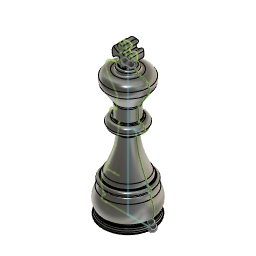
King v1 (Autodesk Fusion 360 design; units mm, degrees)
Autodesk Fusion 360 part; units mm, degrees
sketch "Sketch1" plane through (0, 0, 0) normal (0, 1, 0) x (1, 0, 0)
  spline S0 degree 3 poles (-2.3239, -43.7499) (-1.9635, -43.3416) (-1.5711, -43.0534) (-1.0977, -42.8653) knots 0 0 0 0 1 1 1 1
  spline S1 degree 3 poles (-1.0977, -42.8653) (-0.9162, -42.7932) (-0.7519, -42.7656) (-0.5988, -42.8557) knots 0 0 0 0 1 1 1 1
  spline S2 degree 3 poles (-0.5988, -42.8557) (-0.387, -42.9817) (-0.4437, -43.2144) (-0.4862, -43.3933) knots 0 0 0 0 1 1 1 1
  spline S3 degree 3 poles (-0.4862, -43.3933) (-0.5788, -43.7825) (-0.7682, -44.124) (-1.0818, -44.3926) knots 0 0 0 0 1 1 1 1
  spline S4 degree 3 poles (-1.0818, -44.3926) (-1.35, -44.6225) (-1.2716, -44.7951) (-0.9684, -44.9232) knots 0 0 0 0 1 1 1 1
  spline S5 degree 3 poles (-0.9684, -44.9232) (-0.5113, -45.1159) (-0.0212, -45.1676) (0.4476, -45.1021) knots 0 0 0 0 1 1 1 1
  spline S6 degree 3 poles (0.4476, -45.1021) (1.3114, -44.9807) (1.3468, -44.8256) (0.848, -44.1249) knots 0 0 0 0 1 1 1 1
  spline S7 degree 3 poles (0.848, -44.1249) (0.6019, -43.7791) (0.1882, -43.357) (0.5857, -42.9642) knots 0 0 0 0 1 1 1 1
  spline S8 degree 3 poles (0.5857, -42.9642) (1.0165, -42.5379) (1.4507, -42.9996) (1.7956, -43.2557) knots 0 0 0 0 1 1 1 1
  spline S9 degree 3 poles (1.7956, -43.2557) (2.3849, -43.6932) (2.5622, -43.6807) (2.6819, -42.9725) knots 0 0 0 0 1 1 1 1
  spline S10 degree 3 poles (2.6819, -42.9725) (2.7753, -42.4182) (2.8325, -41.8455) (2.5668, -41.2929) knots 0 0 0 0 1 1 1 1
  spline S11 degree 3 poles (2.5668, -41.2929) (2.4133, -40.9738) (2.3132, -40.8383) (2.0379, -41.1878) knots 0 0 0 0 1 1 1 1
  spline S12 degree 3 poles (2.0379, -41.1878) (1.7877, -41.5044) (1.4382, -41.7092) (1.0528, -41.8168) knots 0 0 0 0 1 1 1 1
  spline S13 degree 3 poles (1.0528, -41.8168) (0.5973, -41.9436) (0.3763, -41.7179) (0.4718, -41.257) knots 0 0 0 0 1 1 1 1
  spline S14 degree 3 poles (0.4718, -41.257) (0.5652, -40.807) (0.8701, -40.4804) (1.1433, -40.1389) knots 0 0 0 0 1 1 1 1
  spline S15 degree 3 poles (1.1433, -40.1389) (1.3568, -39.8719) (1.331, -39.7493) (0.9702, -39.6563) knots 0 0 0 0 1 1 1 1
  spline S16 degree 3 poles (-0.842, -39.6271) (-1.2416, -39.7656) (-1.4835, -39.9145) (-1.0451, -40.3378) knots 0 0 0 0 1 1 1 1
  spline S17 degree 3 poles (-1.0451, -40.3378) (-0.8024, -40.5722) (-0.6643, -40.9205) (-0.5012, -41.2291) knots 0 0 0 0 1 1 1 1
  spline S18 degree 3 poles (-0.5012, -41.2291) (-0.4137, -41.3951) (-0.4491, -41.5836) (-0.5747, -41.7225) knots 0 0 0 0 1 1 1 1
  spline S19 degree 3 poles (-0.5747, -41.7225) (-0.7056, -41.8677) (-0.8674, -41.8681) (-1.0539, -41.7888) knots 0 0 0 0 1 1 1 1
  spline S20 degree 3 poles (-1.0539, -41.7888) (-1.4343, -41.627) (-1.8321, -41.5044) (-2.1103, -41.1678) knots 0 0 0 0 1 1 1 1
  spline S21 degree 3 poles (-2.1103, -41.1678) (-2.3314, -40.9004) (-2.474, -41.0022) (-2.562, -41.2804) knots 0 0 0 0 1 1 1 1
  spline S22 degree 3 poles (-2.562, -41.2804) (-2.8227, -42.1058) (-2.8648, -42.9133) (-2.3239, -43.7499) knots 0 0 0 0 1 1 1 1
  spline S23 degree 3 poles (5.7912, -10.8328) (5.8309, -11.2607) (5.5652, -11.6023) (5.3888, -11.9368) knots 0 0 0 0 1 1 1 1
  spline S24 degree 3 poles (5.3888, -11.9368) (3.7392, -15.0636) (2.7616, -18.3765) (2.5151, -21.9046) knots 0 0 0 0 1 1 1 1
  spline S25 degree 3 poles (2.5151, -21.9046) (2.4513, -22.82) (2.4329, -22.9965) (1.829, -23.074) knots 0 0 0 0 1 1 1 1
  spline S26 degree 3 poles (-2.4465, -23.074) (-2.5929, -23.0336) (-2.7093, -22.9377) (-2.7105, -22.7053) knots 0 0 0 0 1 1 1 1
  spline S27 degree 3 poles (-2.7105, -22.7053) (-2.7118, -22.3537) (-2.8273, -22.0076) (-2.834, -21.6718) knots 0 0 0 0 1 1 1 1
  spline S28 degree 3 poles (-2.834, -21.6718) (-2.8707, -19.8429) (-3.2556, -18.0758) (-3.6952, -16.3157) knots 0 0 0 0 1 1 1 1
  spline S29 degree 3 poles (-3.6952, -16.3157) (-4.1136, -14.6415) (-4.9444, -13.1288) (-5.5825, -11.541) knots 0 0 0 0 1 1 1 1
  spline S30 degree 3 poles (-5.5825, -11.541) (-5.6889, -11.2765) (-5.8736, -11.01) (-5.6901, -10.8328) knots 0 0 0 0 1 1 1 1
  spline S31 degree 3 poles (6.366, -9.2437) (6.6016, -9.3409) (6.7555, -9.5569) (6.8002, -9.828) knots 0 0 0 0 1 1 1 1
  spline S32 degree 3 poles (6.8002, -9.828) (6.8594, -10.1917) (6.5028, -10.4661) (6.102, -10.5763) knots 0 0 0 0 1 1 1 1
  spline S33 degree 3 poles (6.102, -10.5763) (6.0519, -10.5904) (5.9789, -10.5842) (5.9155, -10.5959) knots 0 0 0 0 1 1 1 1
  spline S34 degree 3 poles (-5.9775, -10.5959) (-5.9883, -10.5946) (-5.9996, -10.5942) (-6.0109, -10.5934) knots 0 0 0 0 1 1 1 1
  spline S35 degree 3 poles (-6.0109, -10.5934) (-6.4855, -10.5642) (-6.7612, -10.2876) (-6.7478, -9.8372) knots 0 0 0 0 1 1 1 1
  spline S36 degree 3 poles (-6.7478, -9.8372) (-6.737, -9.4914) (-6.5443, -9.3062) (-6.2461, -9.2437) knots 0 0 0 0 1 1 1 1
  spline S37 degree 3 poles (6.5778, -2.1049) (6.8669, -2.1729) (7.0758, -2.3423) (7.2439, -2.6838) knots 0 0 0 0 1 1 1 1
  spline S38 degree 3 poles (7.2439, -2.6838) (8.1119, -4.4448) (7.8479, -6.1373) (6.9599, -7.7785) knots 0 0 0 0 1 1 1 1
  spline S39 degree 3 poles (6.9599, -7.7785) (6.7297, -8.2039) (6.6129, -8.7857) (6.1437, -9.0068) knots 0 0 0 0 1 1 1 1
  spline S40 degree 3 poles (-2.7568, -9.0068) (-3.2202, -8.9926) (-3.6831, -8.9843) (-4.1428, -9.0068) knots 0 0 0 0 1 1 1 1
  line L0 (-4.1428, -9.0068) -> (-5.7452, -9.0068)
  spline S41 degree 3 poles (-5.7452, -9.0068) (-6.4004, -8.847) (-6.8692, -8.4024) (-7.2763, -7.6358) knots 0 0 0 0 1 1 1 1
  spline S42 degree 3 poles (-7.2763, -7.6358) (-8.1884, -5.9179) (-8.2602, -4.275) (-7.4014, -2.5525) knots 0 0 0 0 1 1 1 1
  spline S43 degree 3 poles (-7.4014, -2.5525) (-7.2792, -2.306) (-7.1278, -2.1675) (-6.9247, -2.1049) knots 0 0 0 0 1 1 1 1
  spline S44 degree 3 poles (-6.9426, -1.8693) (-7.5245, -1.7588) (-7.914, -1.2391) (-7.8143, -0.5701) knots 0 0 0 0 1 1 1 1
  spline S45 degree 3 poles (-7.8143, -0.5701) (-7.7167, 0.0906) (-7.1353, -0.3253) (-6.7766, -0.2389) knots 0 0 0 0 1 1 1 1
  spline S46 degree 3 poles (-6.7766, -0.2389) (-6.6736, -0.2131) (-6.5589, -0.2335) (-6.4492, -0.2335) knots 0 0 0 0 1 1 1 1
  spline S47 degree 3 poles (-6.4492, -0.2335) (-2.0686, -0.2322) (2.3128, -0.2264) (6.6938, -0.2464) knots 0 0 0 0 1 1 1 1
  spline S48 degree 3 poles (6.6938, -0.2464) (6.9666, -0.2477) (7.3691, -0.0512) (7.528, -0.4012) knots 0 0 0 0 1 1 1 1
  spline S49 degree 3 poles (7.528, -0.4012) (7.6906, -0.7586) (7.4992, -1.1227) (7.3102, -1.4572) knots 0 0 0 0 1 1 1 1
  spline S50 degree 3 poles (7.3102, -1.4572) (7.1684, -1.7079) (6.9774, -1.8205) (6.7543, -1.8693) knots 0 0 0 0 1 1 1 1
  spline S51 degree 3 poles (6.0999, -34.4728) (6.4285, -35.0642) (6.4552, -35.692) (6.2659, -36.3197) knots 0 0 0 0 1 1 1 1
  spline S52 degree 3 poles (6.2659, -36.3197) (5.9318, -37.4258) (5.0426, -37.988) (3.7179, -37.9513) knots 0 0 0 0 1 1 1 1
  spline S53 degree 3 poles (3.7179, -37.9513) (3.1649, -37.9354) (2.679, -37.9717) (2.7165, -38.7141) knots 0 0 0 0 1 1 1 1
  spline S54 degree 3 poles (2.7165, -38.7141) (2.7353, -39.0887) (2.4713, -39.2292) (2.1835, -39.23) knots 0 0 0 0 1 1 1 1
  spline S55 degree 3 poles (2.1835, -39.23) (0.7237, -39.235) (-0.7361, -39.2063) (-2.1963, -39.1975) knots 0 0 0 0 1 1 1 1
  spline S56 degree 3 poles (-2.1963, -39.1975) (-2.5629, -39.195) (-2.9366, -39.087) (-2.9495, -38.7137) knots 0 0 0 0 1 1 1 1
  spline S57 degree 3 poles (-2.9495, -38.7137) (-2.9716, -38.0731) (-3.2319, -37.8887) (-3.825, -37.9972) knots 0 0 0 0 1 1 1 1
  spline S58 degree 3 poles (-3.825, -37.9972) (-4.0114, -38.0318) (-4.2162, -37.9746) (-4.411, -37.9542) knots 0 0 0 0 1 1 1 1
  spline S59 degree 3 poles (-4.411, -37.9542) (-6.5343, -37.7336) (-7.162, -35.752) (-6.1794, -34.102) knots 0 0 0 0 1 1 1 1
  spline S60 degree 3 poles (-6.1794, -34.102) (-5.3281, -32.6731) (-4.3413, -31.3251) (-3.4129, -29.9421) knots 0 0 0 0 1 1 1 1
  spline S61 degree 3 poles (-3.4129, -29.9421) (-3.2715, -29.7315) (-3.231, -29.5079) (-3.2473, -29.2543) knots 0 0 0 0 1 1 1 1
  spline S62 degree 3 poles (-3.2473, -29.2543) (-3.3132, -28.2487) (-3.3741, -27.2436) (-3.4133, -26.2372) knots 0 0 0 0 1 1 1 1
  spline S63 degree 3 poles (-3.4133, -26.2372) (-3.4204, -26.0591) (-3.4437, -25.9227) (-3.5092, -25.8251) knots 0 0 0 0 1 1 1 1
  line L1 (-3.5092, -25.8251) -> (-4.0781, -25.8251)
  spline S64 degree 3 poles (-4.0781, -25.8251) (-4.7726, -25.8251) (-5.3356, -25.2625) (-5.3356, -24.5684) knots 0 0 0 0 1 1 1 1
  spline S65 degree 3 poles (-5.3356, -24.5684) (-5.3356, -23.9378) (-4.8714, -23.4177) (-4.2666, -23.3268) knots 0 0 0 0 1 1 1 1
  spline S66 degree 3 poles (-4.2666, -23.3268) (-4.2479, -23.3222) (-4.2308, -23.3155) (-4.212, -23.3114) knots 0 0 0 0 1 1 1 1
  line L2 (-4.212, -23.3114) -> (-4.0781, -23.3114)
  line L3 (3.7338, -23.3114) -> (3.9056, -23.3114)
  spline S67 degree 3 poles (3.9056, -23.3114) (4.1555, -23.3593) (4.3632, -23.4552) (4.5237, -23.5912) knots 0 0 0 0 1 1 1 1
  spline S68 degree 3 poles (4.5237, -23.5912) (4.5287, -23.5946) (4.5333, -23.5987) (4.5383, -23.6025) knots 0 0 0 0 1 1 1 1
  spline S69 degree 3 poles (4.5383, -23.6025) (4.555, -23.6175) (4.5721, -23.6317) (4.5875, -23.6475) knots 0 0 0 0 1 1 1 1
  spline S70 degree 3 poles (4.5875, -23.6475) (4.8353, -23.8769) (4.9909, -24.2039) (4.9909, -24.5684) knots 0 0 0 0 1 1 1 1
  spline S71 degree 3 poles (4.9909, -24.5684) (4.9909, -25.2625) (4.4278, -25.8251) (3.7338, -25.8251) knots 0 0 0 0 1 1 1 1
  line L4 (3.7338, -25.8251) -> (3.275, -25.8251)
  spline S72 degree 3 poles (3.275, -25.8251) (3.2262, -25.8872) (3.1995, -25.9727) (3.1949, -26.0924) knots 0 0 0 0 1 1 1 1
  spline S73 degree 3 poles (3.1949, -26.0924) (3.1511, -27.2557) (3.1098, -28.4189) (3.0535, -29.5813) knots 0 0 0 0 1 1 1 1
  spline S74 degree 3 poles (3.0535, -29.5813) (3.0427, -29.804) (3.1553, -29.9458) (3.2625, -30.1135) knots 0 0 0 0 1 1 1 1
  spline S75 degree 3 poles (3.2625, -30.1135) (4.193, -31.5762) (5.2557, -32.9538) (6.0999, -34.4728) knots 0 0 0 0 1 1 1 1
  line L5 (-0.0015, -0.232) -> (-0.0015, -39.219)
  line L6 (6.5778, -2.1049) -> (6.5778, -1.8693)
  line L7 (6.7543, -1.8693) -> (6.5778, -1.8693)
  line L8 (-0.0015, -0.232) -> (6.6938, -0.2464)
  spline S76 degree 5 poles (6.6938, -0.2464) (6.7066, -0.2449) (6.7318, -0.2418) (6.7681, -0.2374) (6.8135, -0.232) (6.8652, -0.226) (6.9123, -0.2207) (6.9552, -0.2159) (6.9947, -0.2114) (7.0321, -0.2068) (7.0689, -0.2018) (7.1064, -0.1966) (7.1457, -0.1917) (7.1875, -0.1884) (7.2317, -0.189) (7.2778, -0.1954) (7.3248, -0.2096) (7.3716, -0.2326) (7.4166, -0.264) (7.4583, -0.3027) (7.4952, -0.3469) (7.5262, -0.3946) (7.5507, -0.4443) (7.5686, -0.4951) (7.5806, -0.5469) (7.5874, -0.5998) (7.5898, -0.6544) (7.5884, -0.7113) (7.5832, -0.7711) (7.5739, -0.8341) (7.5601, -0.9006) (7.5413, -0.9706) (7.5173, -1.0436) (7.4882, -1.1189) (7.4546, -1.1955) (7.4173, -1.2719) (7.3772, -1.3466) (7.3354, -1.4184) (7.2926, -1.4858) (7.2493, -1.5478) (7.2057, -1.6038) (7.1618, -1.6534) (7.1176, -1.6964) (7.0732, -1.733) (7.0286, -1.7635) (6.9846, -1.7887) (6.9419, -1.8092) (6.9013, -1.8259) (6.8638, -1.8393) (6.8299, -1.8502) (6.8001, -1.8588) (6.7796, -1.864) (6.7662, -1.867) (6.7581, -1.8686) (6.7543, -1.8693) knots 0 0 0 0 0 0 0.02 0.04 0.06 0.08 0.1 0.12 0.14 0.16 0.18 0.2 0.22 0.24 0.26 0.28 0.3 0.32 0.34 0.36 0.38 0.4 0.42 0.44 0.46 0.48 0.5 0.52 0.54 0.56 0.58 0.6 0.62 0.64 0.66 0.68 0.7 0.72 0.74 0.76 0.78 0.8 0.82 0.84 0.86 0.88 0.9 0.92 0.94 0.96 0.98 1 1 1 1 1 1
  line L9 (6.1437, -9.0068) -> (6.1437, -9.2437)
  line L10 (6.366, -9.2437) -> (6.1437, -9.2437)
  line L11 (5.7912, -10.8328) -> (5.7912, -10.5959)
  line L12 (5.7912, -10.5959) -> (5.9155, -10.5959)
  line L13 (1.829, -23.074) -> (1.829, -23.3114)
  line L14 (1.829, -23.3114) -> (3.9056, -23.3114)
  spline S77 degree 5 poles (0.3317, -39.5277) (0.3354, -39.523) (0.3435, -39.5135) (0.3574, -39.499) (0.3799, -39.4788) (0.4148, -39.4523) (0.4572, -39.4245) (0.5074, -39.3951) (0.5659, -39.3642) (0.632, -39.3318) (0.7052, -39.2981) (0.7689, -39.2702) (0.8194, -39.2487) (0.8543, -39.2342) (0.8721, -39.2269) knots 0 0 0 0 0 0 0.1 0.2 0.3 0.4 0.5 0.6 0.7 0.8 0.9 1 1 1 1 1 1
  spline S78 degree 5 poles (-0.3849, -39.5204) (-0.3908, -39.5163) (-0.4031, -39.508) (-0.4234, -39.4949) (-0.4541, -39.4764) (-0.4986, -39.4515) (-0.55, -39.4245) (-0.6088, -39.3954) (-0.675, -39.364) (-0.7484, -39.3306) (-0.8284, -39.2952) (-0.8971, -39.2655) (-0.9512, -39.2425) (-0.9883, -39.2269) (-1.0072, -39.2189) knots 0 0 0 0 0 0 0.1 0.2 0.3 0.4 0.5 0.6 0.7 0.8 0.9 1 1 1 1 1 1
  line L15 (-0.8541, -39.6313) -> (-0.7381, -39.5939)
  spline S79 degree 5 poles (-0.3849, -39.5204) (-0.3903, -39.5208) (-0.4017, -39.5217) (-0.4201, -39.5235) (-0.4471, -39.5272) (-0.4852, -39.5336) (-0.5276, -39.542) (-0.5739, -39.5523) (-0.6234, -39.5643) (-0.675, -39.5776) (-0.7273, -39.592) (-0.7785, -39.6069) (-0.8274, -39.6219) (-0.8728, -39.6367) (-0.9139, -39.6511) (-0.9504, -39.665) (-0.976, -39.6756) (-0.9932, -39.6833) (-1.0037, -39.6883) (-1.0088, -39.6907) knots 0 0 0 0 0 0 0.066667 0.133333 0.2 0.266667 0.333333 0.4 0.466667 0.533333 0.6 0.666667 0.733333 0.8 0.866667 0.933333 1 1 1 1 1 1
  spline S80 degree 5 poles (0.3317, -39.5277) (0.3343, -39.5278) (0.3403, -39.5282) (0.3515, -39.5292) (0.371, -39.5317) (0.403, -39.5365) (0.4427, -39.543) (0.4898, -39.5513) (0.5432, -39.5612) (0.6015, -39.5724) (0.6628, -39.5847) (0.725, -39.5976) (0.7863, -39.611) (0.8451, -39.6244) (0.9007, -39.6378) (0.9525, -39.6511) (0.9909, -39.6616) (1.018, -39.6694) (1.0353, -39.6746) (1.0437, -39.6771) knots 0 0 0 0 0 0 0.066667 0.133333 0.2 0.266667 0.333333 0.4 0.466667 0.533333 0.6 0.666667 0.733333 0.8 0.866667 0.933333 1 1 1 1 1 1
  arc A0 (-1.0223, -39.2078) -> (-1.0072, -39.2189) centre (-0.9916, -39.1819) ccw
  point P0 (6.9525, -0.2161)
  point P1 (7.1237, -0.1946)
  point P2 (7.3297, -0.2138)
  point P3 (7.5889, -0.6614)
  point P4 (7.528, -1.0095)
  point P5 (7.0706, -1.7333)
  point P6 (6.8711, -1.8365)
  point P7 (0.5, -39.4)
  point P8 (-0.6, -39.4)
  point P9 (-0.5713, -39.5519)
  point P10 (-0.8296, -39.6228)
  point P11 (0.4794, -39.5496)
  point P12 (0.7812, -39.61)
  constraint coincident S55 L5.end
  constraint vertical L5
  constraint coincident S48 P0
  constraint coincident S48 P1
  constraint coincident S48 P2
  constraint coincident S49 P3
  constraint coincident S49 P4
  constraint coincident S50 P5
  constraint coincident S50 P6
  constraint coincident S55 S77.end
  constraint coincident S16 L15.start
  constraint coincident S16 S79.end
  constraint coincident S15 S80.end
  constraint coincident S55 A0.start
  constraint tangent S78 A0
revolve "Revolve1" add sketch "Sketch1" angle 360 about axis through (-0.0015, 0, 0.232) along (0, 0, 1) contours S23 S24 S25 S31 S32 S33 S37 S38 S39 S48 S49 S50 S51 S52 S53 S54 S55 L3 S67 S68 S69 S70 S71 L4 S72 S73 S74 S75 L5 L6 L7 L8 S76 L9 L10 L11 L12 L13 L14
extrude "Extrude1" cut sketch "Sketch1" along normal mid plane 4 contours S0 S1 S2 S3 S4 S5 S6 S7 S8 S9 S10 S11 S12 S13 S14 S15 S16 S17 S18 S19 S20 S21 S22 S55 S77 S78 L15 S79 S80 A0
extrude "Extrude2" add sketch "Sketch1" along normal mid plane 4 contours S0 S1 S2 S3 S4 S5 S6 S7 S8 S9 S10 S11 S12 S13 S14 S15 S16 S17 S18 S19 S20 S21 S22 S55 S77 S78 L15 S79 S80 A0
sketch "Sketch2" plane through (0, 0, 25.8251) normal (0, 0, 1) x (-1, 0, 0)
  circle A0 centre (0.0015, 0) radius 3.7353
  circle A1 centre (0.0015, 0) radius 3.2765
  circle A2 centre (0, 0) radius 3.5073 construction
  circle A3 centre (0.0011, -3.5073) radius 0.1
  dimension "d6" = 0.2
  constraint coincident A2.centre origin
  constraint coincident A2 A3.centre
  measures "d6" diameter of A3
extrude "Extrude3" add sketch "Sketch2" along normal blind 0.2 contours A3
pattern_circular "C-Pattern1" count 12 over 360 about axis through (-0.0015, 0, 25.8251) along (0, 0, 1) of "Extrude3"
